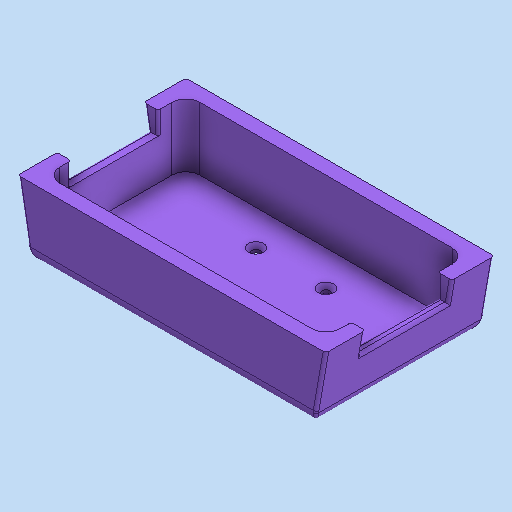
# Autodesk Inventor part: лоток для маркеров
Saved by Autodesk Inventor 2025 (Build 290162000, 162)
## iProperties
Created: 2025-03-03
Part Number: лоток для маркеров
Material: Типовые
Document SubType Name: Modeling
Designer: volko
Density: 1 g/cm^3
Appearance: По умолчанию
Author: volko
Autodesk Inventor part; units mm, degrees
ref_plane "YZ Plane" through (0, 0, 0) normal (1, 0, 0) x (0, 1, 0)
ref_plane "XZ Plane" through (0, 0, 0) normal (0, 1, 0) x (-1, 0, 0)
ref_plane "XY Plane" through (0, 0, 0) normal (0, 0, 1) x (1, 0, 0)
sketch "Эскиз1" plane through (0, 0, 0) normal (0, 1, 0) x (-1, 0, 0)
  line L0 (100, 50) -> (-100, 50)
  line L1 (-100, 50) -> (-100, -50)
  line L2 (-100, -50) -> (100, -50)
  line L3 (100, -50) -> (100, 50)
  line L4 (110, 60) -> (-110, 60)
  line L5 (-110, 60) -> (-110, -60)
  line L6 (-110, -60) -> (110, -60)
  line L7 (110, -60) -> (110, 60)
  line L8 (154, 0) -> (-154, 0) projected
  line L9 (0, -84) -> (0, 84) projected
  point P0 (0, 0)
  point P1 (0, -60)
  point P2 (0, -50)
  point P3 (0, 50)
  point P4 (0, 60)
  dimension "d1" = 220
  dimension "d2" = 10
  dimension "d3" = 10
  dimension "d4" = 120
  constraints: 16 end point, 4 parallel, 2 horizontal, 2 perpendicular, 4 other
  measures "d1" distance of L4.start L4.end
  measures "d2" distance between parallel lines of L7 L3
  measures "d3" distance between parallel lines of L4 L0
  measures "d4" distance of L4.end L5.end
extrude "Выдавливание1" add sketch "Эскиз1" along normal blind 50 contours L0 L9 L4 L7 L8 L3 | L0 L1 L8 L5 L4 L9 | L8 L7 L6 L9 L2 L3 | L1 L2 L9 L6 L5 L8
extrude "Выдавливание2" add sketch "Эскиз1" along normal blind 5
draft "НаклГрань1" angle 10 pull direction (0, -1, 0) faces at (110, 16.6667, 20) (-110, 16.6667, -20) fixed edges at (110, 50, 0) (-110, 50, 0)
sketch "Эскиз4" plane through (0, 0, 0) normal (1, 0, 0) x (0, 1, 0)
  line L0 (50, -50) -> (50, 50) projected
  line L1 (50, 32) -> (34, 32)
  line L2 (34, 32) -> (34, -30)
  line L3 (34, -30) -> (50, -30)
  line L4 (50, 32) -> (50, -30)
  point P0 (0, 0)
  constraints: 8 end point, 2 perpendicular, 2 point on line, 1 collinear, 1 horizontal
extrude "Выдавливание3" cut sketch "Эскиз4" along normal through all both and the other way through all
fillet "Сопряжение1" radius 10 8 edges at (-100, 27.5, 50) (-100, 27.5, -50) (100, 27.5, -50) (100, 27.5, 50) (0, 0, 60) (0, 0, -60) (101.1837, 0, 0) (-101.1837, 0, 0)
fillet "Сопряжение2" radius 2 23 edges at (100, 42, -30) (100, 42, 32) (100, 34, 1) (107.1788, 34, 1) (108.5894, 42, 32) (108.5894, 42, -30) (-108.5894, 42, -30) (-107.1788, 34, 1) (-100, 42, -30) (-108.5894, 42, 32) (-100, 42, 32) (-102.7932, 9.1284, 59.9619) (-99.2205, 2.3396, 56.4279) (-106.4735, 30, 60) (-102.7932, 9.1284, -59.9619) (-99.2205, 2.3396, -56.4279) (-106.4735, 30, -60) (102.7932, 9.1284, -59.9619) (99.2205, 2.3396, -56.4279) (106.4735, 30, -60) (102.7932, 9.1284, 59.9619) (99.2205, 2.3396, 56.4279) (106.4735, 30, 60)
sketch "Эскиз5" plane through (0, 5, 0) normal (0, 1, 0) x (1, 0, 0)
  line L0 (0, 84) -> (0, -84) projected
  line L1 (-154, 0) -> (154, 0) projected
  point P0 (0, 0)
  point P1 (-25, 25)
  point P2 (25, 25)
  point P3 (25, -25)
  point P4 (-25, -25)
  dimension "d31" = 25
  dimension "d32" = 25
  constraints: 4 symmetric about line
  measures "d31" distance from line of L1 point (-25, 25)
  measures "d32" distance from line of point (25, 25) L0
hole "Отверстие1" at (-25, 5, -25) at (25, 5, -25) at (25, 5, 25) at (-25, 5, 25) direction (0, -1, 0) diameter 5.5 end through all countersink diameter 11 countersink angle 90
